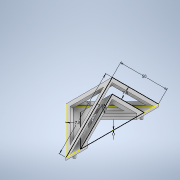
# Autodesk Inventor part: coltar5mmV3
Saved by Autodesk Inventor 2020 (Build 240168000, 168)
## iProperties
Created: 2022-02-13
Part Number: coltar5mmV3
Material: Generic
Document SubType Name: Modeling
Designer: Vlasciar
Density: 1 g/cm^3
Appearance: Default
Author: Vlasciar
Autodesk Inventor part; units mm, degrees
ref_plane "YZ Plane" through (0, 0, 0) normal (1, 0, 0) x (0, 1, 0)
ref_plane "XZ Plane" through (0, 0, 0) normal (0, 1, 0) x (-1, 0, 0)
ref_plane "XY Plane" through (0, 0, 0) normal (0, 0, 1) x (1, 0, 0)
sketch "Sketch2" plane through (0, 0, 0) normal (0, 1, 0) x (-1, 0, 0)
  line L0 (0, 35.355) -> (35.3557, 0)
  line L1 (35.3557, 0) -> (0, -35.355)
  line L2 (0, -35.355) -> (0, 35.355)
  point P0 (0, 0)
  point P1 (0, 0)
  dimension "d1" = 50
  dimension "d41" = 70.71
  constraints: 6 end point, 1 coincident, 1 equal length, 1 horizontal alignment, 1 midpoint
  measures "d1" distance of L0.start L0.end
  measures "d41" distance of L1.end L0.start
extrude "Extrusion1" add sketch "Sketch2" against normal blind 2
sketch "Sketch3" plane through (0, 0, 0) normal (0, 1, 0) x (1, 0, 0)
  line L0 (-35.3557, 0) -> (0, -35.355) projected
  line L1 (0, -35.355) -> (0, 35.355) projected
  line L2 (0, 35.355) -> (-35.3557, 0) projected
  point P0 (0, 0)
sketch "Sketch12" plane through (0, 0, 35.355) normal (1, 0, 0) x (0, 0, -1)
  line L0 (0, 0) -> (70.71, 0) projected
  line L1 (0, 0) -> (35.355, 35.3557)
  line L2 (35.355, 35.3557) -> (70.71, 0)
  line L3 (11.0308, 0) -> (59.6792, 0)
  line L4 (59.6792, 0) -> (35.355, 24.3247)
  line L5 (35.355, 24.3247) -> (11.0308, 0)
  point P0 (35.355, 0)
  point P1 (11.0308, 0)
  point P2 (59.6792, 0)
  dimension "d42" = 50
  dimension "d43" = 50
  dimension "d46" = 0
  dimension "d47" = 7.8
  dimension "d48" = 7.8
  constraints: 10 end point, 2 parallel, 1 horizontal
  measures "d42" distance of L1.end L0.end
  measures "d43" distance of L0.start L1.end
  measures "d46" distance between parallel lines of L0 L3
  measures "d47" distance between parallel lines of L2 L4
  measures "d48" distance between parallel lines of L1 L5
ref_plane "Work Plane5" through (-35.3557, 0, 0) normal (-0.5773466, 0.5773466, 0.5773577) x (0.7071136, 0, 0.7071)
ref_plane "Work Plane6" through (0, 0, -35.355) normal (0.5773466, -0.5773466, 0.5773577) x (-0.7071136, 0, 0.7071)
extrude "Extrusion10" add sketch "Sketch12" along normal up to surface surface through (-35.3557, 0, 0) normal (-0.5773466, 0.5773466, 0.5773577)
split "Split3" plane through (0, 0, -35.355) removes the side toward (-0.5773466, 0.5773466, -0.5773577)
shell "Shell3" thickness 2 removed faces 1 at (0, 11.7852, 0)
sketch "Sketch13" plane through (0, 0, 31.8909) normal (0, 1, 0) x (1, 0, 0)
  line L0 (-31.8916, 31.8909) -> (0, 0) projected
  line L1 (0, 63.7819) -> (0, 0) projected
  line L2 (0, 63.7819) -> (-31.8916, 31.8909) projected
  line L3 (0, 67.2459) -> (0, -3.4641) projected
  line L4 (0, 7.5667) -> (-24.3247, 31.8909)
  line L5 (-24.3247, 31.8909) -> (0, 56.2152)
  line L6 (0, -3.4641) -> (-35.3557, 31.8909) projected
  line L7 (-35.3557, 31.8909) -> (0, 67.2459) projected
  point P0 (0, 31.8909)
  dimension "d52" = 7.8
  dimension "d53" = 7.8
  constraints: 4 end point, 2 parallel, 2 point on line
  measures "d52" distance between parallel lines of L4 L6
  measures "d53" distance between parallel lines of L7 L5
sketch "Sketch19" plane through (0, -2, 0) normal (0, -1, 0) x (1, 0, 0)
  circle A0 centre (-3.6588, 25.1048) radius 1
  line L0 (-2.1113, -27.6684) -> (-27.669, -2.1113) projected
  circle A1 centre (-3.6588, -26.121) radius 1
  line L1 (0, 0) -> (-35.3557, 0) projected
  circle A2 centre (-28.5731, 0) radius 1
  dimension "d79" = 2
  dimension "d80" = 2
  dimension "d81" = 2
  constraints: 3 centre point, 2 point on line
  measures "d79" diameter of A0
  measures "d80" diameter of A1
  measures "d81" diameter of A2
extrude "Extrusion17" add sketch "Sketch19" along normal blind 5
draft "FaceDraft2" angle 10 pull direction (0, -1, 0) faces at (-27.586, -5.3333, -0.1604) (-4.4582, -5.3333, -26.7217) (-2.7103, -5.3333, 24.7881) fixed edges at (-29.5731, -7, 0) (-4.6588, -7, -26.121) (-4.6588, -7, 25.1048)
ref_plane "Work Plane9" through (0, 24.3247, 0) normal (0.5773466, -0.5773466, -0.5773577) x (0, -0.7071136, 0.7071)
ref_plane "Work Plane10" through (0, 0, -24.3242) normal (-0.5773466, 0.5773466, -0.5773577) x (0, 0.7071136, 0.7071)
extrude "Extrusion18" add sketch "Sketch12" against normal up to surface separate body contours L5 L4 L0 surface through (0, 0, -24.3242) normal (-0.5773466, 0.5773466, -0.5773577)
split "Split5" plane through (0, 24.3247, 0) removes the side toward (-0.5773466, 0.5773466, 0.5773577) bodies 2
shell "Shell5" thickness 2 removed faces 1 at (0, 8.1082, 0) bodies 2
sketch "Sketch20" plane through (0, 2, 18.8602) normal (0, 1, 0) x (1, 0, 0)
  line L0 (0, 0) -> (-18.8606, 18.8602) projected
  line L1 (0, 37.7204) -> (0, 0) projected
  line L2 (-18.8606, 18.8602) -> (0, 37.7204) projected
  point P0 (0, 18.8602)
extrude "Extrusion19" cut sketch "Sketch20" against normal blind 10 bodies 2 1
sketch "Sketch21" plane through (-18.8606, 2, 0) normal (0.5773466, -0.5773466, 0.5773577) x (0.4082535, -0.4082535, -0.8164914)
  line L0 (0, 0) -> (0, 26.6729) projected
  line L1 (0, 0) -> (23.0991, 13.3364) projected
  line L2 (0, 26.6729) -> (23.0991, 13.3364) projected
  line L3 (4, 6.9282) -> (4, 19.7446)
  line L4 (4, 19.7446) -> (15.0992, 13.3364)
  line L5 (15.0992, 13.3364) -> (4, 6.9282)
  point P0 (8.5164, 11.9222)
  dimension "d90" = 4
  dimension "d91" = 4
  dimension "d92" = 4
  constraints: 6 end point, 3 parallel
  measures "d90" distance between parallel lines of L0 L3
  measures "d91" distance between parallel lines of L2 L4
  measures "d92" distance between parallel lines of L1 L5
extrude "Extrusion20" cut sketch "Sketch21" against normal blind 2 contours L3 L4 L5 bodies 2
sketch "Sketch22" plane through (-18.8606, 2, 0) normal (0.5773466, -0.5773466, -0.5773577) x (-0.4082535, 0.4082535, -0.8164914)
  line L0 (-23.0991, 13.3364) -> (0, 26.6729) projected
  line L1 (-23.0991, 13.3364) -> (0, 0) projected
  line L2 (0, 0) -> (0, 26.6729) projected
  line L3 (-15.0992, 13.3364) -> (-4, 6.9282)
  line L4 (-4, 6.9282) -> (-4, 19.7446)
  line L5 (-4, 19.7446) -> (-15.0992, 13.3364)
  point P0 (-8.5164, 11.9222)
  dimension "d95" = 4
  dimension "d96" = 4
  dimension "d97" = 4
  constraints: 6 end point, 3 parallel
  measures "d95" distance between parallel lines of L0 L5
  measures "d96" distance between parallel lines of L2 L4
  measures "d97" distance between parallel lines of L1 L3
extrude "Extrusion21" cut sketch "Sketch22" against normal blind 2 contours L5 L4 L3 bodies 2
sketch "Sketch23" plane through (0, 0, 35.355) normal (-0.5773466, 0.5773466, 0.5773577) x (0.8164992, 0.4082418, 0.4082496)
  line L0 (0, 50) -> (-43.3015, 24.9995) projected
  line L1 (-43.3015, 24.9995) -> (0, 0) projected
  line L2 (0, 50) -> (0, 0) projected
  line L3 (-35.3015, 24.9996) -> (-4, 6.9281)
  line L4 (-6.734, 11.6635) -> (-29.8333, 24.9995) projected
  line L5 (-4, 6.9281) -> (-4, 43.0718)
  line L6 (-4, 43.0718) -> (-35.3015, 24.9996)
  point P0 (-14.4337, 24.9995)
  dimension "d100" = 4
  dimension "d101" = 4
  dimension "d102" = 4
  constraints: 6 end point, 4 parallel
  measures "d100" distance between parallel lines of L0 L6
  measures "d101" distance between parallel lines of L1 L3
  measures "d102" distance between parallel lines of L2 L5
extrude "Extrusion22" cut sketch "Sketch23" against normal blind 2 contours L6 L5 L3 bodies 1
sketch "Sketch24" plane through (-35.3557, 0, 0) normal (-0.5773466, 0.5773466, -0.5773577) x (-0.4082535, 0.4082535, 0.8164914)
  line L0 (-43.3011, 25.0002) -> (0, 0) projected
  line L1 (0, 50.0005) -> (0, 0) projected
  line L2 (-43.3011, 25.0002) -> (0, 50.0005) projected
  line L3 (-35.3012, 25.0002) -> (-4, 6.9282)
  line L4 (-4, 6.9282) -> (-4, 43.0722)
  line L5 (-4, 43.0722) -> (-35.3012, 25.0002)
  point P0 (-14.4341, 25.0002)
  dimension "d105" = 4
  dimension "d106" = 4
  dimension "d107" = 4
  constraints: 6 end point, 3 parallel
  measures "d105" distance between parallel lines of L1 L4
  measures "d106" distance between parallel lines of L0 L3
  measures "d107" distance between parallel lines of L2 L5
extrude "Extrusion23" cut sketch "Sketch24" against normal blind 2 contours L5 L4 L3 bodies 1
body "Solid1"
body "Solid4"
